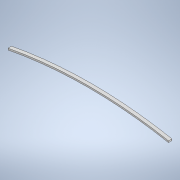
# Autodesk Inventor part: arc_de_cercle
Saved by Autodesk Inventor 2020.2 (Build 242310000, 310)
## iProperties
Created: 2020-01-28
Part Number: arc_de_cercle
Material: Générique
Document SubType Name: Modeling
Designer: anton
Density: 1 g/cm^3
Appearance: Par défaut
Author: anton
Autodesk Inventor part; units mm, degrees
ref_plane "YZ Plane" through (0, 0, 0) normal (1, 0, 0) x (0, 1, 0)
ref_plane "XZ Plane" through (0, 0, 0) normal (0, 1, 0) x (-1, 0, 0)
ref_plane "XY Plane" through (0, 0, 0) normal (0, 0, 1) x (1, 0, 0)
sketch "Esquisse1" plane through (0, 0, 0) normal (0, 0, 1) x (1, 0, 0)
  line L0 (-150.5839, 785.7) -> (150.5839, 785.7)
  arc A0 (150.5839, 785.7) -> (-150.5839, 785.7) centre (0, 0) ccw
  line L1 (-150.5839, 782.7) -> (150.5839, 782.7)
  line L2 (0, 797) -> (-150.5839, 797)
  arc A1 (150.5839, 782.7) -> (-150.5839, 782.7) centre (0, -3) ccw
  line L3 (-150.5839, 785.7) -> (-150.5839, 782.7)
  line L4 (150.5839, 785.7) -> (150.5839, 782.7)
  point P0 (0, 0)
  dimension "d4" = 785.7
  dimension "d8" = 3
  dimension "d9" = 14.3
  constraints: 10 end point, 5 point on circle, 3 horizontal, 2 centre point, 1 perpendicular
  measures "d4" distance from line of point (0, 0) L0
  measures "d8" distance between parallel lines of L0 L1
  measures "d9" distance between parallel lines of L1 L2
extrude "Extrusion1" add sketch "Esquisse1" along normal blind 6.5 contours A0 L2 A1 L0 | L0 A1 L3 | A0 L0 A1 L2 | L0 L4 A1
